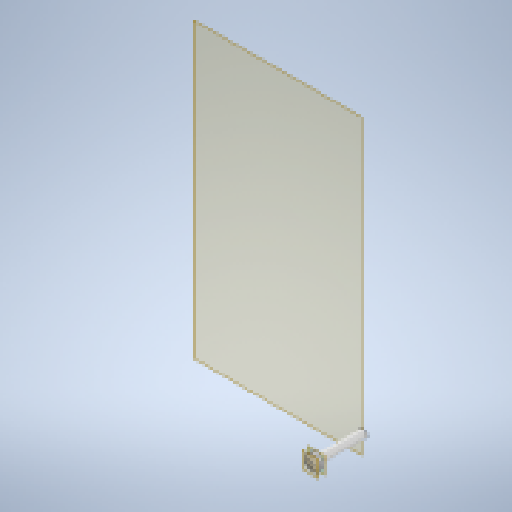
# Autodesk Inventor part: screw
Saved by Autodesk Inventor 2023 (Build 270158000, 158)
## iProperties
Created: 2023-03-12
Part Number: screw
Material: Generic
Document SubType Name: Modeling
Designer: shrey
Density: 1 g/cm^3
Appearance: Default
Author: shrey
Autodesk Inventor part; units mm, degrees
ref_plane "YZ Plane" through (0, 0, 0) normal (1, 0, 0) x (0, 1, 0)
ref_plane "XZ Plane" through (0, 0, 0) normal (0, 1, 0) x (-1, 0, 0)
ref_plane "XY Plane" through (0, 0, 0) normal (0, 0, 1) x (1, 0, 0)
ref_plane "Work Plane1" through (29.0854, -74.8946, 2) normal (0, 0, 1) x (1, 0, 0)
sketch "Sketch1" plane through (29.0854, -74.8946, 2) normal (0, 0, 1) x (1, 0, 0)
  line L0 (19.0856, -32.3111) -> (19.0856, -42.3111) projected
  line L1 (29.0856, -32.3111) -> (19.0856, -32.3111) projected
  line L2 (29.0856, -42.3111) -> (29.0856, -32.3111) projected
  line L3 (19.0856, -42.3111) -> (29.0856, -42.3111) projected
  circle A0 centre (32.6545, -45.7111) radius 1.45
  point P0 (-29.0854, 74.8946)
  dimension "d1" = 2.9
  constraints: 1 centre point
  measures "d1" diameter of A0
extrude "Extrusion1" add sketch "Sketch1" along normal blind 17.9 contours A0
sketch "Sketch2" plane through (61.7399, -120.6057, 19.9) normal (0, 0, 1) x (1, 0, 0)
  circle A0 centre (0, 0) radius 1.45 projected
  circle A1 centre (0, 0) radius 2.915
  point P0 (-61.7399, 120.6057)
  dimension "d4" = 5.83
  constraints: 1 centre point, 1 coincident
  measures "d4" diameter of A1
extrude "Extrusion2" add sketch "Sketch2" along normal blind 1.35 contours A0 | A1
ref_plane "Work Plane2" through (61.7399, -120.6057, 22.26) normal (0, 0, 1) x (1, 0, 0)
sketch "Sketch3" plane through (61.7399, -120.6057, 22.26) normal (0, 0, 1) x (1, 0, 0)
  circle A0 centre (0, 0) radius 1.45 construction
  circle A1 centre (0, 0) radius 1.1446
  point P0 (-61.7399, 120.6057)
  constraints: 1 centre point, 1 coincident
loft "Loft1" add profiles "Sketch3" section 1 edges at (58.8249, -120.6057, 21.25)
ref_plane "Work Plane3" through (61.7399, -120.6057, 19.9) normal (0, 0, -1) x (-1, 0, 0)
body "Solid1"
